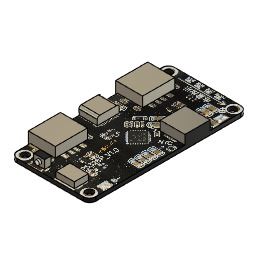
IP5328P (Autodesk Fusion 360 design; units mm, degrees)
Autodesk Fusion 360 part; units mm, degrees
sketch "Sketch1" plane through (0, 0, 0) normal (0, 1, 0) x (1, 0, 0)
  line L0 (0, 0) -> (32.4, 0)
  line L1 (32.4, 0) -> (32.4, 64.8)
  line L2 (32.4, 64.8) -> (0, 64.8)
  line L3 (0, 64.8) -> (0, 0)
  dimension "d1" = 64.8
  dimension "d2" = 32.4
  constraint horizontal L0
  constraint vertical L1
  constraint horizontal L2
  constraint vertical L3
  constraint coincident L0.start L3.end
  measures "d1" distance of L0.end L1.end
  measures "d2" distance of L0.start L0.end
extrude "Extrude1" add sketch "Sketch1" along normal blind 1.62
fillet "Fillet1" radius 2.6 4 edges at (0, 0.81, 0) (32.4, 0.81, 0) (0, 0.81, -64.8) (32.4, 0.81, -64.8)
sketch "Sketch2" plane through (0, 1.62, 0) normal (0, 1, 0) x (-1, 0, 0)
  circle A0 centre (-3, -3) radius 1.5
  circle A1 centre (-29.4, -3) radius 1.5
  circle A2 centre (-29.4, -61.8) radius 1.5
  circle A3 centre (-3, -61.8) radius 1.5
  line L0 (-29.8, -64.8) -> (-2.6, -64.8)
  line L1 (0, -62.2) -> (0, -2.6)
  line L2 (-32.4, -2.6) -> (-32.4, -62.2)
  line L3 (-2.6, 0) -> (-29.8, 0)
  dimension "d6" = 3
  dimension "d7" = 3
  dimension "d8" = 3
  dimension "d9" = 3
  dimension "d10" = 3
  constraint equal A2 A3
  constraint equal A1 A3
  constraint equal A0 A3
  constraint horizontal A0.centre A1.centre
  constraint vertical A0.centre A3.centre
  constraint vertical A1.centre A2.centre
  constraint horizontal A2.centre A3.centre
  measures "d6" diameter of A3
  measures "d7" distance of A3.centre L0
  measures "d8" distance of A3.centre L1
  measures "d9" distance of A2.centre L2
  measures "d10" distance of A1.centre L3
extrude "Extrude2" cut sketch "Sketch2" against normal blind 5
sketch "Sketch3" plane through (0, 0, 0) normal (0, -1, 0) x (1, 0, 0)
  line L0 (10.33, -57.1) -> (-0.77, -57.1)
  line L1 (-0.77, -57.1) -> (-0.77, -43.9)
  line L2 (-0.77, -43.9) -> (10.33, -43.9)
  line L3 (10.33, -43.9) -> (10.33, -57.1)
  line L4 (10.33, -21.2) -> (-0.77, -21.2)
  line L5 (-0.77, -21.2) -> (-0.77, -8)
  line L6 (-0.77, -8) -> (10.33, -8)
  line L7 (10.33, -8) -> (10.33, -21.2)
  line L8 (29.8, -64.8) -> (2.6, -64.8)
  line L9 (2.6, 0) -> (29.8, 0)
  line L10 (0, -62.2) -> (0, -2.6)
  dimension "d13" = 13.2
  dimension "d14" = 11.1
  dimension "d15" = 7.7
  dimension "d16" = 8
  dimension "d17" = 0.77
  constraint horizontal L0
  constraint vertical L1
  constraint horizontal L2
  constraint vertical L3
  constraint horizontal L4
  constraint vertical L5
  constraint horizontal L6
  constraint vertical L7
  constraint vertical L1.end L4.end
  constraint vertical L2.end L4.start
  constraint equal L3 L7
  measures "d13" distance of L0.start L2.end
  measures "d14" distance of L1.end L2.end
  measures "d15" distance of L0 L8
  measures "d16" distance of L6 L9
  measures "d17" distance of L5 L10
extrude "Extrude3" add sketch "Sketch3" against normal blind 5.73
sketch "Sketch4" plane through (0, 1.62, 0) normal (0, 1, 0) x (-1, 0, 0)
  line L0 (-22.2, -39.25) -> (-32.4, -39.25)
  line L1 (-32.4, -39.25) -> (-32.4, -49.6)
  line L2 (-32.4, -49.6) -> (-22.2, -49.6)
  line L3 (-22.2, -49.6) -> (-22.2, -39.25)
  line L4 (-29.8, -64.8) -> (-2.6, -64.8)
  point P0 (-32.4, -62.2)
  dimension "d20" = 10.35
  dimension "d21" = 10.2
  dimension "d22" = 15.2
  constraint horizontal L0
  constraint vertical L1
  constraint horizontal L2
  constraint vertical L3
  constraint vertical L1.end P0
  measures "d20" distance of L0.end L1.end
  measures "d21" distance of L0.start L0.end
  measures "d22" distance of L2 L4
extrude "Extrude4" add sketch "Sketch4" along normal blind 3.8
sketch "Sketch5" plane through (0, 1.62, 0) normal (0, 1, 0) x (-1, 0, 0)
  line L0 (-7.43, -37.16) -> (0.17, -37.16)
  line L1 (0.17, -37.16) -> (0.17, -28.16)
  line L2 (0.17, -28.16) -> (-7.43, -28.16)
  line L3 (-7.43, -28.16) -> (-7.43, -37.16)
  line L4 (0, -43.9) -> (0, -21.2)
  line L5 (-10.33, -43.9) -> (0, -43.9)
  dimension "d25" = 9
  dimension "d26" = 7.6
  dimension "d27" = 0.17
  dimension "d28" = 6.74
  constraint horizontal L0
  constraint vertical L1
  constraint horizontal L2
  constraint vertical L3
  measures "d25" distance of L0.start L2.end
  measures "d26" distance of L0.start L0.end
  measures "d27" distance of L1 L4
  measures "d28" distance of L0 L5
extrude "Extrude5" add sketch "Sketch5" along normal blind 3.2
fillet "Fillet2" radius 1 4 edges at (-0.085, 1.62, -28.16) (3.63, 4.82, -28.16) (3.63, 4.82, -37.16) (-0.085, 1.62, -37.16)
sketch "Sketch6" plane through (0, 1.62, 0) normal (0, 1, 0) x (-1, 0, 0)
  line L0 (-7.68, -4.38) -> (-12.18, -4.38)
  line L1 (-12.18, -4.38) -> (-12.18, -1.73)
  line L2 (-12.18, -1.73) -> (-7.68, -1.73)
  line L3 (-7.68, -1.73) -> (-7.68, -4.38)
  line L4 (-2.6, 0) -> (-29.8, 0)
  line L5 (0, -8) -> (0, -2.6)
  dimension "d32" = 4.5
  dimension "d33" = 2.65
  dimension "d34" = 1.73
  dimension "d35" = 7.68
  constraint horizontal L0
  constraint vertical L1
  constraint horizontal L2
  constraint vertical L3
  measures "d32" distance of L0.start L0.end
  measures "d33" distance of L0.end L1.end
  measures "d34" distance of L2 L4
  measures "d35" distance of L3 L5
extrude "Extrude6" add sketch "Sketch6" along normal blind 3.5
sketch "Sketch7" plane through (0, 0, -1.73) normal (0, 0, 1) x (1, 0, 0)
  circle A0 centre (9.93, 3.31) radius 0.95
  line L0 (7.68, 5.12) -> (12.18, 5.12)
  point P0 (9.93, 5.12)
  dimension "d38" = 1.9
  dimension "d39" = 1.81
  constraint midpoint L0 P0
  constraint vertical A0.centre P0
  measures "d38" diameter of A0
  measures "d39" distance of A0.centre L0
extrude "Extrude7" add sketch "Sketch7" along normal blind 0.86
sketch "Sketch8" plane through (0, 1.62, 0) normal (0, 1, 0) x (-1, 0, 0)
  line L0 (-17.54, -6.8) -> (-25.14, -6.8)
  line L1 (-25.14, -6.8) -> (-25.14, -1)
  line L2 (-25.14, -1) -> (-17.54, -1)
  line L3 (-17.54, -1) -> (-17.54, -6.8)
  line L4 (-2.6, 0) -> (-29.8, 0)
  line L5 (-32.4, -2.6) -> (-32.4, -39.25)
  dimension "d42" = 5.8
  dimension "d43" = 7.6
  dimension "d44" = 1
  dimension "d45" = 7.26
  constraint horizontal L0
  constraint vertical L1
  constraint horizontal L2
  constraint vertical L3
  measures "d42" distance of L0.start L2.end
  measures "d43" distance of L0.start L0.end
  measures "d44" distance of L2 L4
  measures "d45" distance of L1 L5
extrude "Extrude8" add sketch "Sketch8" along normal blind 2.42
equation "d7 = 1.5 mm + d6 / 2"
equation "d8 = d7"
equation "d9 = d7"
equation "d10 = d7"
equation "d18 = -1 * ( 4.11 mm + 1.62 mm )"
equation "d39 = 0.86 mm + d38 / 2"
